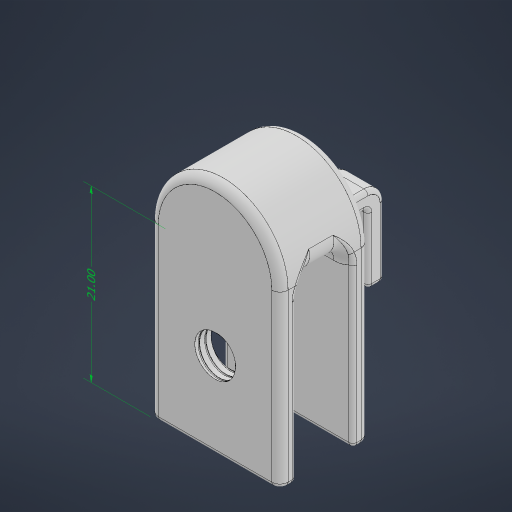
# Autodesk Inventor part: 부품1
Saved by Autodesk Inventor 2024 (Build 280153000, 153)
## iProperties
Created: 2024-01-30
Part Number: 부품1
Material: 일반
Document SubType Name: Modeling
Designer: KBU
Density: 1 g/cm^3
Appearance: 기본값
Author: KBU
Autodesk Inventor part; units mm, degrees
ref_plane "YZ Plane" through (0, 0, 0) normal (1, 0, 0) x (0, 1, 0)
ref_plane "XZ Plane" through (0, 0, 0) normal (0, 1, 0) x (-1, 0, 0)
ref_plane "XY Plane" through (0, 0, 0) normal (0, 0, 1) x (1, 0, 0)
sketch "스케치1" plane through (0, 0, 0) normal (0, 0, 1) x (1, 0, 0)
  line L0 (-2.35, -5.3) -> (2.35, -5.3)
  line L1 (2.35, -5.3) -> (2.35, 5.3)
  line L2 (2.35, 5.3) -> (-2.35, 5.3)
  line L3 (-2.35, 5.3) -> (-2.35, -5.3)
  line L4 (-2.35, -5.3) -> (2.35, 5.3) construction
  line L5 (2.35, -5.3) -> (-2.35, 5.3) construction
  line L6 (-2.35, 3.3) -> (2.35, 3.3)
  point P0 (0, 0)
  dimension "d0" = 10.6
  dimension "d1" = 4.7
  dimension "d2" = 2
  constraints: 14 end point, 2 horizontal, 2 midpoint, 2 parallel, 2 point on line, 1 perpendicular
  measures "d0" distance of L0.end L1.end
  measures "d1" distance of L1.end L2.end
  measures "d2" distance between parallel lines of L2 L6
extrude "돌출1" add sketch "스케치1" against normal blind 2
extrude "돌출2" add sketch "스케치1" along normal blind 5.5 contours L3 L2 L1 L6
sketch "스케치2" plane through (0, 0, 5.5) normal (0, 0, 1) x (1, 0, 0)
  line L0 (2.35, 5.3) -> (-2.35, 5.3) projected
  arc A0 (8, 5.3) -> (-8, 5.3) centre (0, 5.3) ccw
  line L1 (-8, 5.3) -> (-8, -15.7)
  line L2 (-8, -15.7) -> (8, -15.7)
  line L3 (8, -15.7) -> (8, 5.3)
  point P0 (0, 0)
  dimension "d7" = 16
  dimension "d8" = 21
  dimension "d9" = 8
  constraints: 6 end point, 2 perpendicular, 2 point on circle, 1 centre point, 1 midpoint, 1 tangent, 1 vertical
  measures "d7" diameter of A0
  measures "d8" distance of L1.start L1.end
  measures "d9" distance from line of L3 point (0, 0)
extrude "돌출3" add sketch "스케치2" along normal blind 2
sketch "스케치3" plane through (0, 0, 7.5) normal (0, 0, 1) x (1, 0, 0)
  arc A0 (8, 5.3) -> (-8, 5.3) centre (0, 5.3) ccw projected
  line L0 (-8, 5.3) -> (8, 5.3)
  point P0 (0, 0)
  constraints: 2 end point, 1 horizontal
extrude "돌출4" add sketch "스케치3" along normal blind 9
sketch "스케치4" plane through (0, 0, 16.5) normal (0, 0, 1) x (1, 0, 0)
  line L0 (-8, 5.3) -> (8, 5.3) projected
  line L1 (8, -15.7) -> (8, 5.3) projected
  line L2 (-8, 5.3) -> (8, 5.3)
  line L3 (8, 5.3) -> (8, -15.7)
  line L4 (8, -15.7) -> (-8, -15.7)
  line L5 (-8, -15.7) -> (-8, 5.3)
  point P0 (0, 0)
  constraints: 8 end point, 2 parallel, 1 horizontal, 1 perpendicular
extrude "돌출5" add sketch "스케치4" against normal blind 2
fillet "모깎기1" radius 0.5 7 edges at (0, 3.3, 0) (0, -5.3, 0) (0, -5.3, -2) (0, 3.3, 5.5) (-2.35, 4.3, 5.5) (0, 5.3, 5.5) (2.35, 4.3, 5.5)
fillet "모깎기2" radius 2 1 edges at (0, 5.3, -2)
fillet "모깎기3" radius 0.5 22 edges at (-2.4964, 3.1536, 5.3536) (-2.35, 3.1536, 0.1464) (-2.35, -1, 0) (-2.35, -5.1536, -0.1464) (-2.35, -5.3, -1) (-2.35, -5.1536, -1.8536) (-2.35, -0.75, -2) (-2.35, 4.7142, -1.4142) (-2.35, 5.3, 2.5) (-2.4964, 5.4464, 5.3536) (-2.35, 3.3, 2.75) (2.35, -5.1536, -1.8536) (2.35, -5.3, -1) (2.35, -5.1536, -0.1464) (2.35, -1, 0) (2.35, 3.1536, 0.1464) (2.35, 3.3, 2.75) (2.4964, 3.1536, 5.3536) (2.35, 4.7142, -1.4142) (2.35, 5.3, 2.5) (2.4964, 5.4464, 5.3536) (2.35, -0.75, -2)
fillet "모깎기6" radius 2 2 edges at (-8, 5.3, 11) (8, 5.3, 11)
fillet "모깎기7" radius 2 6 edges at (0, 5.3, 14.5) (-7.2898, 6.1453, 14.5) (7.2898, 6.1453, 14.5) (0, 5.3, 7.5) (-7.2898, 6.1453, 7.5) (7.2898, 6.1453, 7.5)
fillet "모깎기8" radius 0.5 12 edges at (8, 4.6873, 7.5611) (8, -5.8209, 7.5) (7.8609, 6.7852, 8.5079) (7.8609, 6.7852, 13.4921) (8, -5.8209, 14.5) (8, 4.6873, 14.4389) (-8, 4.6873, 14.4389) (-8, -5.8209, 14.5) (-7.8609, 6.7852, 13.4921) (-8, 4.6873, 7.5611) (-8, -5.8209, 7.5) (-7.8609, 6.7852, 8.5079)
fillet "모깎기9" radius 1 6 edges at (0, 13.3, 5.5) (8, -5.2, 5.5) (-8, -5.2, 5.5) (0, 13.3, 16.5) (8, -5.2, 16.5) (-8, -5.2, 16.5)
fillet "모깎기10" radius 0.5 16 edges at (0, -15.7, 16.5) (7.7071, -15.7, 16.2071) (8, -15.7, 15.25) (7.8536, -15.7, 14.6464) (0, -15.7, 14.5) (-7.8536, -15.7, 14.6464) (-8, -15.7, 15.25) (-7.7071, -15.7, 16.2071) (7.8536, -15.7, 7.3536) (8, -15.7, 6.75) (7.7071, -15.7, 5.7929) (0, -15.7, 5.5) (-7.7071, -15.7, 5.7929) (-8, -15.7, 6.75) (-7.8536, -15.7, 7.3536) (0, -15.7, 7.5)
sketch "스케치5" plane through (0, 0, 16.5) normal (0, 0, 1) x (1, 0, 0)
  line L0 (1.85, 2.8) -> (1.85, -4.8) projected
  line L1 (-7, -15.7) -> (7, -15.7) projected
  circle A0 centre (0, -5.2) radius 2.5
  point P0 (0, 0)
  dimension "d31" = 10.5
  dimension "d32" = 5
  constraints: 1 centre point
  measures "d31" distance from line of L1 A0.centre
  measures "d32" diameter of A0
extrude "돌출6" cut sketch "스케치5" against normal blind 2
sketch "스케치6" plane through (0, 0, 0) normal (1, 0, 0) x (0, 1, 0)
  line L0 (-5.2, 0.2744) -> (-5.2, 26.8584)
  line L1 (-2.7, 16.5) -> (-2.7, 14.5) projected
  line L2 (-2.45, 16.5) -> (-2.45, 14.5)
  line L3 (-7.7, 16.5) -> (-7.7, 14.5) projected
  line L4 (-3.2196, 17) -> (-3.2196, 16.2)
  line L5 (-3.2196, 16.2) -> (-2.5268, 16.6)
  line L6 (-2.5268, 16.6) -> (-3.2196, 17)
  line L7 (-3.133, 16.95) -> (-3.133, 16.25) construction
  line L8 (-2.96, 16.8501) -> (-2.96, 16.3499) construction
  line L9 (-2.7, 16.7) -> (-2.7, 16.5) construction
  arc A0 (-2.6567, 16.525) -> (-2.6567, 16.675) centre (-2.7, 16.6) ccw
  point P0 (0, 0)
  dimension "d39" = 2.5
  dimension "d52" = 60
  dimension "d53" = 60
  dimension "d54" = 0.8
  dimension "d55" = 4.134
  dimension "d56" = 4.48
  dimension "d57" = 5
  dimension "d58" = 0.433
  dimension "d61" = 0.6928
  dimension "d62" = 0.0866
  dimension "d63" = 0.1732
  dimension "d64" = 0
  constraints: 16 end point, 8 point on line, 7 vertical, 2 parallel, 2 point on circle, 1 centre point, 1 coincident, 1 midpoint, 1 tangent, 4 other
  measures "d39" distance between parallel lines of L0 L1
  measures "d52" angle of L6 L4
  measures "d53" angle of L4 L5
  measures "d54" distance of L4.start L4.end
  measures "d55" diameter of L7 L0
  measures "d56" diameter of L8 L0
  measures "d57" diameter of point (-2.7, 16.6) L0
  measures "d58" distance between parallel lines of L9 L7
  measures "d61" distance from line of L5.end L4
  measures "d62" distance between parallel lines of L4 L7
  measures "d63" distance from line of L5.end L9
  measures "d64" distance of L1.start L9.end
coil "코일1" sketch "스케치6" operation cut axis through (0, -5.2, 0.2744) along (0, 0, -1) pitch 0.8 turns 5 hand right contours L6 A0 L5 L4
equation "\"d62\" = 0.125 * d61"
